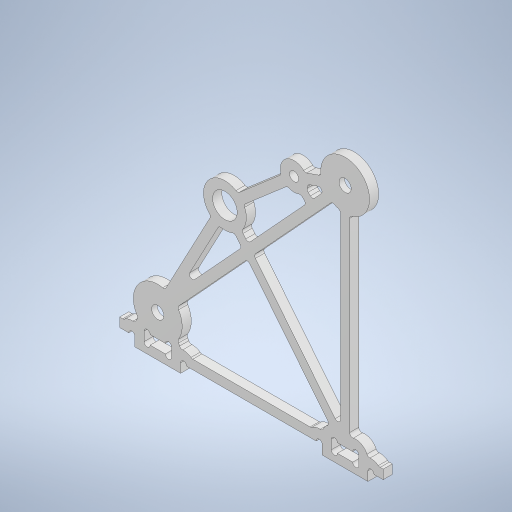
# Autodesk Inventor part: アーム 左フレーム
Saved by Autodesk Inventor 2023 (Build 270158000, 158)
## iProperties
Created: 2020-05-03
Part Number: アーム 左フレーム
Material: アルミニウム 2014-T6
Document SubType Name: Modeling
Designer: mozar
Density: 2.78927 g/cm^3
Appearance: サテン
Mass: 13.4791 g
Surface Area: 59.0115 cm^2
Volume: 4.83249 cm^3
Author: mozar
Autodesk Inventor part; units mm, degrees
(part 1 of 2)
ref_plane "YZ Plane" through (0, 0, 0) normal (1, 0, 0) x (0, 1, 0)
ref_plane "XZ Plane" through (0, 0, 0) normal (0, 1, 0) x (-1, 0, 0)
ref_plane "XY Plane" through (0, 0, 0) normal (0, 0, 1) x (1, 0, 0)
sketch "スケッチ1" plane through (0, 0, 0) normal (0, 0, 1) x (1, 0, 0)
  arc A0 (39.9627, 86.1428) -> (39.4448, 84.9887) centre (40.4104, 85.2486) ccw
  arc A1 (39.7226, 83.6386) -> (39.4448, 84.9887) centre (28.3399, 82) ccw
  arc A2 (39.7226, 83.6386) -> (40.6541, 82.7828) centre (40.7124, 83.7811) ccw
  line L0 (40.6541, 82.7828) -> (57.3541, 81.8067)
  arc A3 (57.3541, 81.8067) -> (58.3494, 82.4556) centre (57.4124, 82.805) ccw
  arc A4 (59.9805, 85.044) -> (58.3494, 82.4556) centre (65.3767, 79.8352) ccw
  arc A5 (59.9805, 85.044) -> (60.1364, 86.2219) centre (59.261, 85.7385) ccw
  line L1 (60.1364, 86.2219) -> (56.2648, 93.2331)
  arc A6 (56.2648, 93.2331) -> (54.9416, 93.6438) centre (55.3894, 92.7497) ccw
  line L2 (54.9416, 93.6438) -> (39.9627, 86.1428)
  arc A7 (62.7626, 87.6721) -> (63.8426, 87.1766) centre (63.638, 88.1555) ccw
  arc A8 (65.8023, 87.3231) -> (63.8426, 87.1766) centre (65.3767, 79.8352) ccw
  arc A9 (65.8023, 87.3231) -> (66.7965, 87.9737) centre (65.859, 88.3215) ccw
  line L3 (66.7965, 87.9737) -> (71.2039, 99.8518)
  arc A10 (71.2039, 99.8518) -> (69.8186, 101.0938) centre (70.2663, 100.1996) ccw
  line L4 (69.8186, 101.0938) -> (59.416, 95.8845)
  arc A11 (59.416, 95.8845) -> (58.9884, 94.5069) centre (59.8638, 94.9903) ccw
  line L5 (58.9884, 94.5069) -> (62.7626, 87.6721)
  arc A12 (68.6447, 103.8611) -> (68.5001, 105.7082) centre (68.197, 104.7553) ccw
  line L6 (68.5001, 105.7082) -> (51.8505, 111.0032)
  arc A13 (51.8505, 111.0032) -> (50.6721, 109.5669) centre (51.5475, 110.0503) ccw
  line L7 (50.6721, 109.5669) -> (56.5694, 98.8874)
  arc A14 (56.5694, 98.8874) -> (57.8925, 98.4767) centre (57.4448, 99.3708) ccw
  line L8 (57.8925, 98.4767) -> (68.6447, 103.8611)
  arc A15 (53.4182, 96.236) -> (53.8458, 97.6136) centre (52.9704, 97.1302) ccw
  line L9 (53.8458, 97.6136) -> (47.1934, 109.6604)
  arc A16 (47.1934, 109.6604) -> (45.4441, 109.6631) centre (46.318, 109.177) ccw
  line L10 (45.4441, 109.6631) -> (35.6044, 91.9739)
  arc A17 (35.6044, 91.9739) -> (35.8272, 90.7287) centre (36.4783, 91.4878) ccw
  arc A18 (37.3851, 89.1018) -> (35.8272, 90.7287) centre (28.3399, 82) ccw
  arc A19 (37.3851, 89.1018) -> (38.6194, 88.8252) centre (38.1716, 89.7194) ccw
  line L11 (38.6194, 88.8252) -> (53.4182, 96.236)
  circle A20 centre (28.3399, 82) radius 7.5
  circle A21 centre (74.8156, 105.2737) radius 1.5
  arc A22 (-14.025, 48) -> (-12.025, 48) centre (-13.025, 48) ccw
  line L12 (-12.025, 48) -> (-12.025, 51)
  arc A23 (-12.025, 51) -> (-14.025, 51) centre (-13.025, 51) ccw
  line L13 (-14.025, 51) -> (-19.025, 51)
  arc A24 (-19.025, 51) -> (-21.025, 51) centre (-20.025, 51) ccw
  line L14 (-21.025, 51) -> (-21.025, 48)
  arc A25 (-21.025, 48) -> (-19.025, 48) centre (-20.025, 48) ccw
  line L15 (-19.025, 48) -> (-14.025, 48)
  arc A26 (60.3767, 48) -> (62.3767, 48) centre (61.3767, 48) ccw
  line L16 (62.3767, 48) -> (62.3767, 51)
  arc A27 (62.3767, 51) -> (60.3767, 51) centre (61.3767, 51) ccw
  line L17 (60.3767, 51) -> (55.3767, 51)
  arc A28 (55.3767, 51) -> (53.3767, 51) centre (54.3767, 51) ccw
  line L18 (53.3767, 51) -> (53.3767, 48)
  arc A29 (53.3767, 48) -> (55.3767, 48) centre (54.3767, 48) ccw
  line L19 (55.3767, 48) -> (60.3767, 48)
  arc A30 (43.4972, 112.3347) -> (43.549, 113.1991) centre (42.6234, 112.8208) ccw
  arc A31 (43.3678, 113.8351) -> (43.549, 113.1991) centre (46.326, 114.3342) ccw
  arc A32 (43.3678, 113.8351) -> (42.8681, 114.5425) centre (42.3817, 113.6687) ccw
  line L20 (42.8681, 114.5425) -> (33.2246, 119.9111)
  arc A33 (33.2246, 119.9111) -> (32.0339, 119.7474) centre (32.7382, 119.0374) ccw
  arc A34 (28.9631, 117.8488) -> (32.0339, 119.7474) centre (26.4001, 125.4272) ccw
  arc A35 (28.9631, 117.8488) -> (28.2844, 116.8569) centre (29.2834, 116.9015) ccw
  line L21 (28.2844, 116.8569) -> (29.2919, 94.3022)
  arc A36 (29.2919, 94.3022) -> (30.1348, 93.3591) centre (30.2909, 94.3468) ccw
  arc A37 (31.8073, 92.9648) -> (30.1348, 93.3591) centre (28.3399, 82) ccw
  arc A38 (31.8073, 92.9648) -> (32.9827, 93.4322) centre (32.1088, 93.9183) ccw
  line L22 (32.9827, 93.4322) -> (43.4972, 112.3347)
  arc A39 (69.6092, 86.93) -> (69.9385, 85.7884) centre (70.5467, 86.5822) ccw
  arc A40 (72.822, 80.7396) -> (69.9385, 85.7884) centre (65.3767, 79.8352) ccw
  arc A41 (72.822, 80.7396) -> (73.638, 79.876) centre (73.8147, 80.8602) ccw
  line L23 (73.638, 79.876) -> (87.0818, 77.4622)
  arc A42 (87.0818, 77.4622) -> (88.1269, 78.9424) centre (87.2585, 78.4465) ccw
  line L24 (88.1269, 78.9424) -> (76.1666, 99.8838)
  arc A43 (76.1666, 99.8838) -> (74.3607, 99.7357) centre (75.2982, 99.3878) ccw
  line L25 (74.3607, 99.7357) -> (69.6092, 86.93)
  arc A44 (73.1078, 76.9232) -> (72.0424, 76.3973) centre (72.9311, 75.9389) ccw
  arc A45 (67.5826, 72.667) -> (72.0424, 76.3973) centre (65.3767, 79.8352) ccw
  arc A46 (67.5826, 72.667) -> (66.8767, 71.7112) centre (67.8767, 71.7112) ccw
  line L26 (66.8767, 71.7112) -> (66.8767, 58.0524)
  arc A47 (66.8767, 58.0524) -> (68.5183, 57.2854) centre (67.8767, 58.0524) ccw
  line L27 (68.5183, 57.2854) -> (87.0165, 72.7581)
  arc A48 (87.0165, 72.7581) -> (86.5516, 74.5094) centre (86.3749, 73.5252) ccw
  line L28 (86.5516, 74.5094) -> (73.1078, 76.9232)
  arc A49 (-29.708, 65.4922) -> (-29.5215, 64.3049) centre (-28.8251, 65.0226) ccw
  arc A50 (-28.6541, 63.3116) -> (-29.5215, 64.3049) centre (-35.0928, 58.5637) ccw
  arc A51 (-28.6541, 63.3116) -> (-27.5026, 62.9671) centre (-27.8492, 63.9051) ccw
  line L29 (-27.5026, 62.9671) -> (-4.985, 71.2866)
  arc A52 (-4.985, 71.2866) -> (-4.395, 72.5749) centre (-5.3316, 72.2246) ccw
  line L30 (-4.395, 72.5749) -> (-11.0543, 90.3814)
  arc A53 (-11.0543, 90.3814) -> (-12.0966, 91.0255) centre (-11.9909, 90.0311) ccw
  arc A54 (-15.1677, 91.227) -> (-12.0966, 91.0255) centre (-13.05, 100) ccw
  arc A55 (-15.1677, 91.227) -> (-16.2852, 90.7245) centre (-15.4023, 90.2549) ccw
  line L31 (-16.2852, 90.7245) -> (-29.708, 65.4922)
  arc A56 (-4.1377, 98.5784) -> (-3.549, 97.5038) centre (-3.1501, 98.4209) ccw
  line L32 (-3.549, 97.5038) -> (17.7068, 88.2599)
  arc A57 (17.7068, 88.2599) -> (18.9244, 88.6028) centre (18.1056, 89.177) ccw
  arc A58 (21.267, 91.0677) -> (18.9244, 88.6028) centre (28.3399, 82) ccw
  arc A59 (21.267, 91.0677) -> (21.5476, 92.3011) centre (20.652, 91.8562) ccw
  line L33 (21.5476, 92.3011) -> (10.495, 114.5492)
  arc A60 (10.495, 114.5492) -> (9.6102, 115.1042) centre (9.5994, 114.1043) ccw
  arc A61 (7.9613, 115.4364) -> (9.6102, 115.1042) centre (9.6587, 119.604) ccw
  arc A62 (7.9613, 115.4364) -> (6.9306, 115.2672) centre (7.5841, 114.5103) ccw
  line L34 (6.9306, 115.2672) -> (-4.721, 105.2086)
  arc A63 (-4.721, 105.2086) -> (-4.9636, 104.0076) centre (-4.0676, 104.4516) ccw
  arc A64 (-4.1377, 98.5784) -> (-4.9636, 104.0076) centre (-13.05, 100) ccw
  circle A65 centre (65.3767, 52.702) radius 1.5
  arc A66 (-24.6969, 51.9865) -> (-27.425, 51.2) centre (-25.025, 48) ccw
  arc A67 (-24.6969, 51.9865) -> (-23.6969, 52.5865) centre (-24.6149, 52.9832) ccw
  arc A68 (-22.7265, 53.9499) -> (-23.6969, 52.5865) centre (-20.025, 51) ccw
  arc A69 (-22.7265, 53.9499) -> (-23.2864, 55.6807) centre (-23.4019, 54.6874) ccw
  line L35 (-23.2864, 55.6807) -> (-26.6781, 56.0751)
  arc A70 (-26.6781, 56.0751) -> (-27.7157, 55.4687) centre (-26.7936, 55.0818) ccw
  arc A71 (-29.6192, 52.7293) -> (-27.7157, 55.4687) centre (-35.0928, 58.5637) ccw
  arc A72 (-29.6192, 52.7293) -> (-28.935, 51) centre (-28.935, 52) ccw
  line L36 (-28.935, 51) -> (-28.025, 51)
  arc A73 (-28.025, 51) -> (-27.425, 51.2) centre (-28.025, 52) ccw
  circle A74 centre (4.1532, 54) radius 1.5
  circle A75 centre (-35.0928, 58.5637) radius 4
  arc A76 (-6.2073, 53.6947) -> (-6.6633, 51.7611) centre (-6.3229, 52.7014) ccw
  arc A77 (-5.625, 51.2) -> (-6.6633, 51.7611) centre (-8.025, 48) ccw
  arc A78 (-5.625, 51.2) -> (-5.025, 51) centre (-5.025, 52) ccw
  line L37 (-5.025, 51) -> (-0.2915, 51)
  arc A79 (-0.2915, 51) -> (-0.176, 52.9933) centre (-0.2915, 52) ccw
  line L38 (-0.176, 52.9933) -> (-6.2073, 53.6947)
  circle A80 centre (-42.5549, 50.4818) radius 1.5
  circle A81 centre (92.0829, 75.0403) radius 1.5
  circle A82 centre (34.927, 132.3764) radius 1.5
  circle A83 centre (26.4001, 125.4272) radius 4
  arc A84 (38.4894, 120.4137) -> (39.8212, 121.8216) centre (38.9758, 121.2874) ccw
  line L39 (39.8212, 121.8216) -> (36.0614, 127.7726)
  arc A85 (36.0614, 127.7726) -> (34.2364, 127.0372) centre (35.216, 127.2385) ccw
  arc A86 (34.1958, 123.6306) -> (34.2364, 127.0372) centre (26.4001, 125.4272) ccw
  arc A87 (34.1958, 123.6306) -> (34.6838, 122.5323) centre (35.1702, 123.406) ccw
  line L40 (34.6838, 122.5323) -> (38.4894, 120.4137)
  circle A88 centre (46.326, 114.3342) radius 1.5
  arc A89 (68.7767, 51.2) -> (68.7327, 51.2326) centre (66.3767, 48) ccw
  arc A90 (68.7767, 51.2) -> (69.3767, 51) centre (69.3767, 52) ccw
  line L41 (69.3767, 51) -> (77.3767, 51)
  arc A91 (77.3767, 51) -> (78.3767, 52) centre (77.3767, 52) ccw
  line L42 (78.3767, 52) -> (78.3767, 59.4801)
  arc A92 (78.3767, 59.4801) -> (76.7351, 60.2472) centre (77.3767, 59.4801) ccw
  line L43 (76.7351, 60.2472) -> (68.7342, 53.5548)
  arc A93 (68.7342, 53.5548) -> (68.376, 52.7664) centre (69.3758, 52.7878) ccw
  arc A94 (68.3354, 52.206) -> (68.376, 52.7664) centre (65.3767, 52.702) ccw
  arc A95 (68.3354, 52.206) -> (68.7327, 51.2326) centre (69.3217, 52.0407) ccw
  arc A96 (-24.7713, 60.778) -> (-24.5402, 58.8467) centre (-24.4247, 59.84) ccw
  line L44 (-24.5402, 58.8467) -> (0.2632, 55.9625)
  arc A97 (0.2632, 55.9625) -> (1.3153, 57.3061) centre (0.3787, 56.9558) ccw
  line L45 (1.3153, 57.3061) -> (-2.6435, 67.8917)
  arc A98 (-2.6435, 67.8917) -> (-3.9267, 68.4794) centre (-3.5802, 67.5414) ccw
  line L46 (-3.9267, 68.4794) -> (-24.7713, 60.778)
  arc A99 (-7.8805, 92.6022) -> (-8.2443, 91.4322) centre (-7.3077, 91.7825) ccw
  line L47 (-8.2443, 91.4322) -> (-1.5781, 73.6072)
  arc A100 (-1.5781, 73.6072) -> (-0.2949, 73.0195) centre (-0.6415, 73.9575) ccw
  line L48 (-0.2949, 73.0195) -> (16.3317, 79.1624)
  arc A101 (16.3317, 79.1624) -> (16.9735, 80.2524) centre (15.9851, 80.1005) ccw
  arc A102 (17.0899, 84.3844) -> (16.9735, 80.2524) centre (28.3399, 82) ccw
  arc A103 (17.0899, 84.3844) -> (16.5104, 85.5088) centre (16.1116, 84.5918) ccw
  line L49 (16.5104, 85.5088) -> (-4.7454, 94.7527)
  arc A104 (-4.7454, 94.7527) -> (-5.9328, 94.4506) centre (-5.1442, 93.8357) ccw
  arc A105 (-7.8805, 92.6022) -> (-5.9328, 94.4506) centre (-13.05, 100) ccw
  arc A106 (18.5677, 75.9375) -> (17.3714, 76.3484) centre (17.718, 75.4104) ccw
  line L50 (17.3714, 76.3484) -> (0.7634, 70.2123)
  arc A107 (0.7634, 70.2123) -> (0.1733, 68.924) centre (1.11, 69.2743) ccw
  line L51 (0.1733, 68.924) -> (4.0811, 58.475)
  arc A108 (4.0811, 58.475) -> (5.7745, 58.1716) centre (5.0177, 58.8253) ccw
  line L52 (5.7745, 58.1716) -> (19.1987, 73.7122)
  arc A109 (19.1987, 73.7122) -> (19.2338, 74.9766) centre (18.4419, 74.3659) ccw
  arc A110 (18.5677, 75.9375) -> (19.2338, 74.9766) centre (28.3399, 82) ccw
  arc A111 (22.7149, 71.9696) -> (21.469, 71.7511) centre (22.2257, 71.0974) ccw
  line L53 (21.469, 71.7511) -> (7.3295, 55.3824)
  arc A112 (7.3295, 55.3824) -> (7.103, 54.5465) centre (8.0862, 54.7287) ccw
  arc A113 (6.7512, 52.5) -> (7.103, 54.5465) centre (4.1532, 54) ccw
  arc A114 (6.7512, 52.5) -> (7.6173, 51) centre (7.6173, 52) ccw
  line L54 (7.6173, 51) -> (25.8399, 51)
  arc A115 (25.8399, 51) -> (26.8399, 52) centre (25.8399, 52) ccw
  line L55 (26.8399, 52) -> (26.8399, 69.7526)
  arc A116 (26.8399, 69.7526) -> (26.0399, 70.7323) centre (25.8399, 69.7526) ccw
  arc A117 (22.7149, 71.9696) -> (26.0399, 70.7323) centre (28.3399, 82) ccw
  arc A118 (30.6399, 70.7323) -> (29.8399, 69.7526) centre (30.8399, 69.7526) ccw
  line L56 (29.8399, 69.7526) -> (29.8399, 52)
  arc A119 (29.8399, 52) -> (30.8399, 51) centre (30.8399, 52) ccw
  line L57 (30.8399, 51) -> (46.3767, 51)
  arc A120 (46.3767, 51) -> (46.9767, 51.2) centre (46.3767, 52) ccw
  arc A121 (49.7048, 51.9865) -> (46.9767, 51.2) centre (49.3767, 48) ccw
  arc A122 (49.7048, 51.9865) -> (50.7048, 52.5865) centre (49.7868, 52.9832) ccw
  arc A123 (56.7767, 54.2) -> (50.7048, 52.5865) centre (54.3767, 51) ccw
  arc A124 (56.7767, 54.2) -> (57.3767, 54) centre (57.3767, 55) ccw
  line L58 (57.3767, 54) -> (58.3767, 54)
  arc A125 (58.3767, 54) -> (58.9767, 54.2) centre (58.3767, 55) ccw
  arc A126 (59.0037, 54.2201) -> (58.9767, 54.2) centre (61.3767, 51) ccw
  arc A127 (59.0037, 54.2201) -> (59.0309, 55.8094) centre (58.4105, 55.0251) ccw
  line L59 (59.0309, 55.8094) -> (37.0148, 73.2252)
  arc A128 (37.0148, 73.2252) -> (35.75, 73.2056) centre (36.3944, 72.4409) ccw
  arc A129 (30.6399, 70.7323) -> (35.75, 73.2056) centre (28.3399, 82) ccw
  arc A130 (25.5394, 93.1538) -> (26.2949, 94.1683) centre (25.2959, 94.1237) ccw
  line L60 (26.2949, 94.1683) -> (25.2874, 116.723)
  arc A131 (25.2874, 116.723) -> (24.5231, 117.6505) centre (24.2884, 116.6784) ccw
  arc A132 (19.8716, 120.8035) -> (24.5231, 117.6505) centre (26.4001, 125.4272) ccw
  arc A133 (19.8716, 120.8035) -> (18.727, 121.17) centre (19.0555, 120.2256) ccw
  line L61 (18.727, 121.17) -> (14.7786, 119.7967)
  arc A134 (14.7786, 119.7967) -> (14.1165, 118.9889) centre (15.1071, 118.8522) ccw
  arc A135 (13.2739, 116.9243) -> (14.1165, 118.9889) centre (9.6587, 119.604) ccw
  arc A136 (13.2739, 116.9243) -> (13.1817, 115.8839) centre (14.0773, 116.3288) ccw
  line L62 (13.1817, 115.8839) -> (24.2343, 93.6359)
  arc A137 (24.2343, 93.6359) -> (25.3867, 93.1143) centre (25.1298, 94.0808) ccw
  arc A138 (25.5394, 93.1538) -> (25.3867, 93.1143) centre (28.3399, 82) ccw
  arc A139 (16.6463, 125.18) -> (18.408, 125.7823) centre (17.409, 125.8267) ccw
  arc A140 (30.493, 132.3009) -> (18.408, 125.7823) centre (26.4001, 125.4272) ccw
  arc A141 (30.493, 132.3009) -> (31.9852, 132.9642) centre (31.0046, 133.1602) ccw
  arc A142 (37.763, 131.3981) -> (31.9852, 132.9642) centre (34.927, 132.3764) ccw
  arc A143 (37.763, 131.3981) -> (37.8629, 130.5378) centre (38.7083, 131.0719) ccw
  line L63 (37.8629, 130.5378) -> (45.9263, 117.7752)
  arc A144 (45.9263, 117.7752) -> (46.6603, 117.3156) centre (46.7717, 118.3093) ccw
  arc A145 (49.126, 115.4113) -> (46.6603, 117.3156) centre (46.326, 114.3342) ccw
  arc A146 (49.126, 115.4113) -> (49.7562, 114.8174) centre (50.0593, 115.7703) ccw
  line L64 (49.7562, 114.8174) -> (72.2946, 107.6495)
  arc A147 (72.2946, 107.6495) -> (73.1521, 107.7703) centre (72.5976, 108.6025) ccw
  arc A148 (77.6052, 104.17) -> (73.1521, 107.7703) centre (74.8156, 105.2737) ccw
  arc A149 (77.6052, 104.17) -> (77.6667, 103.3062) centre (78.5351, 103.8022) ccw
  line L65 (77.6667, 103.3062) -> (91.8368, 78.4957)
  arc A150 (91.8368, 78.4957) -> (92.5496, 78.0038) centre (92.7052, 78.9916) ccw
  arc A151 (91.4896, 72.0996) -> (92.5496, 78.0038) centre (92.0829, 75.0403) ccw
  arc A152 (91.4896, 72.0996) -> (90.6502, 71.8864) centre (91.2918, 71.1193) ccw
  line L66 (90.6502, 71.8864) -> (81.7351, 64.4294)
  arc A153 (81.7351, 64.4294) -> (81.3767, 63.6624) centre (82.3767, 63.6624) ccw
  line L67 (81.3767, 63.6624) -> (81.3767, 48)
  line L68 (81.3767, 48) -> (67.3767, 48)
  arc A154 (67.3767, 48) -> (65.3767, 48) centre (66.3767, 48) ccw
  line L69 (65.3767, 48) -> (65.3767, 45)
  line L70 (65.3767, 45) -> (50.3767, 45)
  line L71 (50.3767, 45) -> (50.3767, 48)
  arc A155 (50.3767, 48) -> (48.3767, 48) centre (49.3767, 48) ccw
  line L72 (48.3767, 48) -> (-7.025, 48)
  arc A156 (-7.025, 48) -> (-9.025, 48) centre (-8.025, 48) ccw
  line L73 (-9.025, 48) -> (-9.025, 45)
  line L74 (-9.025, 45) -> (-24.025, 45)
  line L75 (-24.025, 45) -> (-24.025, 48)
  arc A157 (-24.025, 48) -> (-26.025, 48) centre (-25.025, 48) ccw
  line L76 (-26.025, 48) -> (-40.586, 48)
  arc A158 (-40.586, 48) -> (-41.0782, 47.8705) centre (-40.586, 47) ccw
  arc A159 (-42.9601, 53.4544) -> (-41.0782, 47.8705) centre (-42.5549, 50.4818) ccw
  arc A160 (-42.9601, 53.4544) -> (-42.206, 54.9028) centre (-43.0951, 54.4452) ccw
  arc A161 (-36.1143, 66.4982) -> (-42.206, 54.9028) centre (-35.0928, 58.5637) ccw
  arc A162 (-36.1143, 66.4982) -> (-35.6612, 68.3041) centre (-36.242, 67.49) ccw
  arc A163 (16.6463, 125.18) -> (-35.6612, 68.3041) centre (-13.05, 100) ccw
  arc A164 (58.092, 78.0514) -> (57.179, 78.8118) centre (57.1207, 77.8135) ccw
  line L77 (57.179, 78.8118) -> (40.479, 79.7879)
  arc A165 (40.479, 79.7879) -> (39.4542, 79.0465) centre (40.4207, 78.7896) ccw
  arc A166 (38.6039, 76.8133) -> (39.4542, 79.0465) centre (28.3399, 82) ccw
  arc A167 (38.6039, 76.8133) -> (38.876, 75.578) centre (39.4964, 76.3623) ccw
  line L78 (38.876, 75.578) -> (62.2563, 57.083)
  arc A168 (62.2563, 57.083) -> (63.8767, 57.8673) centre (62.8767, 57.8673) ccw
  line L79 (63.8767, 57.8673) -> (63.8767, 71.7112)
  arc A169 (63.8767, 71.7112) -> (63.1709, 72.667) centre (62.8767, 71.7112) ccw
  arc A170 (58.092, 78.0514) -> (63.1709, 72.667) centre (65.3767, 79.8352) ccw
  circle A171 centre (65.3767, 79.8352) radius 4.5
  arc A172 (-21.9546, 98.5311) -> (-22.8529, 99.3644) centre (-22.9413, 98.3683) ccw
  line L80 (-22.8529, 99.3644) -> (-47.8911, 101.5872)
  arc A173 (-47.8911, 101.5872) -> (-48.9794, 100.608) centre (-47.9795, 100.5911) ccw
  arc A174 (-48.9794, 100.608) -> (-32.1537, 69.5642) centre (-13.05, 100) ccw
  arc A175 (-32.1537, 69.5642) -> (-30.7392, 69.9415) centre (-31.622, 70.4111) ccw
  line L81 (-30.7392, 69.9415) -> (-18.9338, 92.1335)
  arc A176 (-18.9338, 92.1335) -> (-19.1416, 93.341) centre (-19.8166, 92.6031) ccw
  arc A177 (-21.9546, 98.5311) -> (-19.1416, 93.341) centre (-13.05, 100) ccw
  arc A178 (-17.8733, 107.628) -> (-17.4559, 108.78) centre (-18.4077, 108.4732) ccw
  line L82 (-17.4559, 108.78) -> (-25.1673, 132.7046)
  arc A179 (-25.1673, 132.7046) -> (-26.4932, 133.3253) centre (-26.1191, 132.3979) ccw
  arc A180 (-26.4932, 133.3253) -> (-48.5246, 105.731) centre (-13.05, 100) ccw
  arc A181 (-48.5246, 105.731) -> (-47.6258, 104.5754) centre (-47.5374, 105.5715) ccw
  line L83 (-47.6258, 104.5754) -> (-22.5876, 102.3526)
  arc A182 (-22.5876, 102.3526) -> (-21.5566, 103.0147) centre (-22.4992, 103.3487) ccw
  arc A183 (-17.8733, 107.628) -> (-21.5566, 103.0147) centre (-13.05, 100) ccw
  arc A184 (11.2534, 123.8119) -> (12.3137, 125.4554) centre (11.6078, 124.747) ccw
  arc A185 (12.3137, 125.4554) -> (-21.598, 134.903) centre (-13.05, 100) ccw
  arc A186 (-21.598, 134.903) -> (-22.3119, 133.625) centre (-21.3602, 133.9317) ccw
  line L84 (-22.3119, 133.625) -> (-14.6006, 109.7003)
  arc A187 (-14.6006, 109.7003) -> (-13.5891, 109.0089) centre (-13.6488, 110.0071) ccw
  arc A188 (-7.905, 107.4148) -> (-13.5891, 109.0089) centre (-13.05, 100) ccw
  arc A189 (-7.905, 107.4148) -> (-6.6814, 107.4795) centre (-7.3349, 108.2364) ccw
  line L85 (-6.6814, 107.4795) -> (4.9702, 117.5381)
  arc A190 (4.9702, 117.5381) -> (5.288, 118.533) centre (4.3167, 118.295) ccw
  arc A191 (11.2534, 123.8119) -> (5.288, 118.533) centre (9.6587, 119.604) ccw
  circle A192 centre (9.6587, 119.604) radius 1.5
  circle A193 centre (-13.05, 100) radius 4.025
  circle A194 centre (-13.05, 100) radius 7.025
  circle A195 centre (-35.0928, 58.5637) radius 8
  circle A196 centre (26.4001, 125.4272) radius 8
  circle A197 centre (9.6587, 119.604) radius 4.5
  line L86 (-35.0928, 58.5637) -> (-13.05, 100) construction
  line L87 (-33.7685, 57.8592) -> (-11.7257, 99.2955)
  line L88 (-14.3743, 100.7045) -> (-36.4171, 59.2682)
  arc A198 (-36.4171, 59.2682) -> (-33.7685, 57.8592) centre (-35.0928, 58.5637) ccw
  arc A199 (-11.7257, 99.2955) -> (-14.3743, 100.7045) centre (-13.05, 100) ccw
  line L89 (-13.05, 100) -> (9.6587, 119.604) construction
  line L90 (-12.0698, 98.8646) -> (10.6389, 118.4685)
  line L91 (8.6785, 120.7394) -> (-14.0302, 101.1354)
  arc A200 (-14.0302, 101.1354) -> (-12.0698, 98.8646) centre (-13.05, 100) ccw
  arc A201 (10.6389, 118.4685) -> (8.6785, 120.7394) centre (9.6587, 119.604) ccw
  line L92 (9.6587, 119.604) -> (26.4001, 125.4272) construction
  line L93 (10.1515, 118.1872) -> (26.8929, 124.0104)
  line L94 (25.9073, 126.8439) -> (9.1659, 121.0207)
  arc A202 (9.1659, 121.0207) -> (10.1515, 118.1872) centre (9.6587, 119.604) ccw
  arc A203 (26.8929, 124.0104) -> (25.9073, 126.8439) centre (26.4001, 125.4272) ccw
  line L95 (26.4001, 125.4272) -> (-35.0928, 58.5637) construction
  line L96 (25.296, 126.4426) -> (-36.1968, 59.5791)
  line L97 (-33.9887, 57.5483) -> (27.5042, 124.4118)
  arc A204 (27.5042, 124.4118) -> (25.296, 126.4426) centre (26.4001, 125.4272) ccw
  arc A205 (-36.1968, 59.5791) -> (-33.9887, 57.5483) centre (-35.0928, 58.5637) ccw
  point P0 (0, 0)
  point P1 (0, 0)
  point P2 (-24.0714, 79.2818)
  point P3 (-1.6956, 109.802)
  point P4 (18.0294, 122.5156)
  point P5 (-4.3463, 91.9954)
  point P6 (-14.9489, 93.2365)
  point P7 (-6.8748, 103.3493)
  point P8 (6.9306, 115.2672)
  point P9 (7.4274, 115.6961)
  point P10 (7.9613, 115.4364)
  point P11 (13.2739, 116.9243)
  point P12 (14.1586, 119.581)
  point P13 (18.727, 121.17)
  point P14 (19.471, 121.4288)
  point P15 (19.9767, 120.6586)
  point P16 (-28.2664, 68.2022)
  point P17 (5.467, 117.967)
  point P18 (-6.6814, 107.4795)
  point P19 (-8.8352, 105.6202)
  point P20 (-17.5975, 94.6455)
  point P21 (-30.7392, 69.9415)
  point P22 (-32.7265, 66.2057)
  point P23 (-28.6541, 63.3116)
  point P24 (-28.6693, 63.3323)
  point P25 (22.1848, 118.6278)
  point P26 (24.5231, 117.6505)
  point P27 (34.1958, 123.6306)
  point P28 (34.2364, 127.0372)
  point P29 (18.4854, 124.2623)
  point P30 (13.1731, 122.4145)
  dimension "d0" = 3
  dimension "d1" = 3
  dimension "d2" = 3
  dimension "d3" = 3
  dimension "d4" = 3
  constraints: 378 point on circle, 204 end point, 203 centre point, 16 tangent, 15 horizontal, 14 vertical, 4 midpoint, 4 parallel, 3 coincident, 1 concentric, 723 other
  measures "d0" radial gap between concentric circles of A193 A194
  measures "d1" diameter of A199
  measures "d2" diameter of A201
  measures "d3" diameter of A203
  measures "d4" diameter of A205
extrude "押し出し1" add sketch "スケッチ1" against normal blind 3 contours A34 A196 A132 L97 A83 L94 A140 A86 | L97 L62 L96 A132 | A132 L96 L93 A83 L97 | A132 A196 L93 L96 | L97 L33 L96 L62 | L97 A203 L94 A83 | A83 L93 A203 L97 | L96 A83 L93 | L93 A196 L94 A83 L96 | L97 L32 L96 L33 | A83 L96 A204 A203 L93 | L61 L93 A197 L94 A196 | A83 L94 A204 L96 | L97 L49 L96 L32 | A197 A61 L90 L93 A135 | L97 L47 L96 L49 | L94 A192 L91 A197 A191 | A197 L93 L90 A192 L94 | L97 L30 L96 L47 | A195 L88 A75 L97 A50 A71 A161 | A192 | L93 A192 L90 | L90 A197 L91 A192 L93 | L97 A50 A49 L31 L96 L30 | L88 L81 A194 L87 L31 L96 A195 | A195 L96 A75 L88 | L90 L34 A194 L91 L85 A197 | L97 A75 L87 A195 A50 | L96 L31 L87 A195 | A195 L87 A75 L96 | L88 A198 L97 A75 | A75 L96 A205 L88 | A195 L87 A49 | L97 A198 L87 A75 | A75 L87 A198 A205 L96 | L90 A193 L91 A194 | A194 L87 A193 L90 | L88 A193 L87 A194 | A194 L91 A193 L88 | L90 L87 A199 L91 A193 | A193 L87 L90 | L88 A200 L90 L87 A193 | A193 L91 A199 L88 | L90 A200 A199 L87
hole "穴1" at (9.6587, 119.604, 0) direction (0, 0, -1) diameter 3 depth 12 tip angle 118
hole "穴2" at (-13.05, 100, 0) direction (0, 0, -1) diameter 8.05 depth 12 tip angle 118
hole "穴3" at (26.4001, 125.4272, 0) at (-35.0928, 58.5637, 0) direction (0, 0, -1) diameter 4 depth 12 tip angle 118
sketch "スケッチ2" plane through (0, 0, -3) normal (0, 0, -1) x (-1, 0, 0)
  circle A0 centre (-26.4001, 125.4272) radius 2 projected
  circle A1 centre (35.0928, 58.5637) radius 2 projected
  circle A2 centre (13.05, 100) radius 4.025 projected
  circle A3 centre (-9.6587, 119.604) radius 1.5 projected
  arc A4 (6.8748, 103.3493) -> (14.9489, 93.2365) centre (13.05, 100) ccw projected
  line L0 (6.8748, 103.3493) -> (-7.4274, 115.6961) projected
  arc A5 (-14.1586, 119.581) -> (-7.4274, 115.6961) centre (-9.6587, 119.604) ccw projected
  line L1 (-14.1586, 119.581) -> (-19.471, 121.4288) projected
  arc A6 (-19.9767, 120.6586) -> (-19.471, 121.4288) centre (-26.4001, 125.4272) ccw projected
  line L2 (-19.9767, 120.6586) -> (28.2664, 68.2022) projected
  line L3 (28.2664, 68.2022) -> (14.9489, 93.2365) projected
  line L4 (-5.467, 117.967) -> (8.8352, 105.6202) projected
  arc A7 (17.5975, 94.6455) -> (8.8352, 105.6202) centre (13.05, 100) ccw projected
  line L5 (17.5975, 94.6455) -> (32.7265, 66.2057) projected
  arc A8 (28.6693, 63.3323) -> (32.7265, 66.2057) centre (35.0928, 58.5637) ccw projected
  line L6 (28.6693, 63.3323) -> (-22.1848, 118.6278) projected
  arc A9 (-18.4854, 124.2623) -> (-22.1848, 118.6278) centre (-26.4001, 125.4272) ccw projected
  line L7 (-18.4854, 124.2623) -> (-13.1731, 122.4145) projected
  arc A10 (-5.467, 117.967) -> (-13.1731, 122.4145) centre (-9.6587, 119.604) ccw projected
  circle A11 centre (35.0928, 58.5637) radius 4
  circle A12 centre (-26.4001, 125.4272) radius 2 projected
  circle A13 centre (-26.4001, 125.4272) radius 4
  point P0 (0, 0)
  dimension "d28" = 8
  dimension "d29" = 8
  constraints: 2 centre point, 2 coincident
  measures "d28" diameter of A11
  measures "d29" diameter of A13
extrude "押し出し2" cut sketch "スケッチ2" against normal blind 0.7 contours A0 | A1 | A11 | A13
sketch "スケッチ3" plane through (0, 0, -3) normal (0, 0, -1) x (-1, 0, 0)
  circle A0 centre (35.0928, 58.5637) radius 4 projected
  circle A1 centre (-26.4001, 125.4272) radius 4 projected
  circle A2 centre (13.05, 100) radius 4.025 projected
  circle A3 centre (-9.6587, 119.604) radius 1.5 projected
  arc A4 (6.8748, 103.3493) -> (14.9489, 93.2365) centre (13.05, 100) ccw projected
  line L0 (6.8748, 103.3493) -> (-7.4274, 115.6961) projected
  arc A5 (-14.1586, 119.581) -> (-7.4274, 115.6961) centre (-9.6587, 119.604) ccw projected
  line L1 (-14.1586, 119.581) -> (-19.471, 121.4288) projected
  arc A6 (-19.9767, 120.6586) -> (-19.471, 121.4288) centre (-26.4001, 125.4272) ccw projected
  line L2 (-19.9767, 120.6586) -> (28.2664, 68.2022) projected
  line L3 (28.2664, 68.2022) -> (14.9489, 93.2365) projected
  line L4 (-5.467, 117.967) -> (8.8352, 105.6202) projected
  arc A7 (17.5975, 94.6455) -> (8.8352, 105.6202) centre (13.05, 100) ccw projected
  line L5 (17.5975, 94.6455) -> (32.7265, 66.2057) projected
  arc A8 (28.6693, 63.3323) -> (32.7265, 66.2057) centre (35.0928, 58.5637) ccw projected
  line L6 (28.6693, 63.3323) -> (-22.1848, 118.6278) projected
  arc A9 (-18.4854, 124.2623) -> (-22.1848, 118.6278) centre (-26.4001, 125.4272) ccw projected
  line L7 (-18.4854, 124.2623) -> (-13.1731, 122.4145) projected
  arc A10 (-5.467, 117.967) -> (-13.1731, 122.4145) centre (-9.6587, 119.604) ccw projected
  circle A11 centre (13.05, 100) radius 4.025 projected
  line L8 (13.05, 100) -> (5.4504, 93.0108) construction
  line L9 (28.2664, 68.2022) -> (-19.9767, 120.6586) projected
  line L10 (12.0346, 101.1041) -> (4.435, 94.1149)
  line L11 (6.4658, 91.9067) -> (14.0654, 98.8959)
  arc A12 (14.0654, 98.8959) -> (12.0346, 101.1041) centre (13.05, 100) ccw
  arc A13 (4.435, 94.1149) -> (6.4658, 91.9067) centre (5.4504, 93.0108) ccw
  line L12 (-9.6587, 119.604) -> (-14.7232, 114.9463) construction
  line L13 (-10.6741, 120.708) -> (-15.7386, 116.0504)
  line L14 (-13.7078, 113.8422) -> (-8.6433, 118.4999)
  arc A14 (-8.6433, 118.4999) -> (-10.6741, 120.708) centre (-9.6587, 119.604) ccw
  arc A15 (-15.7386, 116.0504) -> (-13.7078, 113.8422) centre (-14.7232, 114.9463) ccw
  point P0 (0, 0)
  point P1 (9.2502, 96.5054)
  point P2 (-12.1909, 117.2751)
  point P3 (9.0139, 94.2502)
  point P4 (6.9831, 96.4583)
  point P5 (-11.7661, 115.6279)
  point P6 (-13.7969, 117.8361)
  dimension "d33" = 3
  dimension "d34" = 3
  constraints: 16 end point, 8 point on circle, 8 tangent, 4 centre point, 2 midpoint, 2 parallel, 2 perpendicular, 2 point on line
  measures "d33" diameter of A13
  measures "d34" diameter of A15
extrude "押し出し3" add sketch "スケッチ3" against normal blind 3 contours L2 L13 A5 L14
fillet "フィレット1" radius 1 19 edges at (22.1848, 118.6278, -1.5) (19.9767, 120.6586, -1.5) (19.471, 121.4288, -1.5) (18.4854, 124.2623, -1.5) (13.1731, 122.4145, -1.5) (14.1586, 119.581, -1.5) (13.7969, 117.8361, -1.5) (15.7386, 116.0504, -1.5) (13.7078, 113.8422, -1.5) (11.7661, 115.6279, -1.5) (7.4274, 115.6961, -1.5) (5.467, 117.967, -1.5) (-6.8748, 103.3493, -1.5) (-8.8352, 105.6202, -1.5) (-14.9489, 93.2365, -1.5) (-17.5975, 94.6455, -1.5) (-28.2664, 68.2022, -1.5) (-32.7265, 66.2057, -1.5) (-28.6693, 63.3323, -1.5)
sketch "スケッチ4" plane through (0, 0, -3) normal (0, 0, -1) x (-1, 0, 0)
  line L0 (9.025, 45) -> (24.025, 45) projected
  line L1 (26.025, 48) -> (40.586, 48) projected
  arc A0 (28.2548, 62.7161) -> (28.1361, 63.912) centre (27.4001, 63.2351) ccw projected
  line L2 (28.1361, 63.912) -> (-21.6516, 118.048) projected
  arc A1 (-21.6516, 118.048) -> (-22.8335, 118.2662) centre (-22.3876, 117.3711) ccw projected
  arc A2 (-18.4115, 125.0013) -> (-22.8335, 118.2662) centre (-26.4001, 125.4272) ccw projected
  arc A3 (-18.4115, 125.0013) -> (-17.7414, 124.0035) centre (-17.4129, 124.948) ccw projected
  line L3 (-17.7414, 124.0035) -> (-13.793, 122.6301) projected
  arc A4 (-13.793, 122.6301) -> (-12.7725, 122.8527) centre (-13.4645, 123.5746) ccw projected
  arc A5 (-5.288, 118.533) -> (-12.7725, 122.8527) centre (-9.6587, 119.604) ccw projected
  arc A6 (-5.288, 118.533) -> (-4.9702, 117.5381) centre (-4.3167, 118.295) ccw projected
  line L4 (-4.9702, 117.5381) -> (8.2579, 106.1185) projected
  arc A7 (8.2579, 106.1185) -> (9.4271, 106.0187) centre (8.9114, 106.8755) ccw projected
  arc A8 (18.1172, 95.1344) -> (9.4271, 106.0187) centre (13.05, 100) ccw projected
  arc A9 (18.1172, 95.1344) -> (17.9557, 93.9721) centre (18.8385, 94.4418) ccw projected
  line L5 (17.9557, 93.9721) -> (32.3566, 66.9011) projected
  arc A10 (32.3566, 66.9011) -> (33.4453, 66.3922) centre (33.2394, 67.3708) ccw projected
  arc A11 (28.2548, 62.7161) -> (33.4453, 66.3922) centre (35.0928, 58.5637) ccw projected
  line L6 (-13.0309, 113.1062) -> (22.9794, 73.9509) projected
  arc A12 (22.9794, 73.9509) -> (24.5983, 75.0975) centre (23.7154, 74.6278) ccw projected
  line L7 (24.5983, 75.0975) -> (15.3071, 92.5632) projected
  arc A13 (15.3071, 92.5632) -> (14.253, 93.0788) centre (14.4242, 92.0935) ccw projected
  arc A14 (-11.2244, 115.3851) -> (-12.2492, 115.1836) centre (-11.5723, 114.4476) ccw projected
  line L8 (-12.2492, 115.1836) -> (-12.9717, 114.5191) projected
  arc A15 (-12.9717, 114.5191) -> (-13.0309, 113.1062) centre (-12.2948, 113.7831) ccw projected
  arc A16 (6.5669, 102.7056) -> (6.2975, 103.8477) centre (5.644, 103.0907) ccw projected
  line L9 (6.2975, 103.8477) -> (-6.9306, 115.2672) projected
  arc A17 (-6.9306, 115.2672) -> (-7.9613, 115.4364) centre (-7.5841, 114.5103) ccw projected
  arc A18 (-11.2244, 115.3851) -> (-7.9613, 115.4364) centre (-9.6587, 119.604) ccw projected
  arc A19 (-17.4982, 120.7426) -> (-18.5628, 119.1212) centre (-17.8267, 119.7981) ccw projected
  arc A20 (-16.4155, 116.7864) -> (-15.0025, 116.7273) centre (-15.6794, 117.4633) ccw projected
  line L10 (-15.0025, 116.7273) -> (-14.28, 117.3918) projected
  arc A21 (-14.28, 117.3918) -> (-13.9936, 118.3962) centre (-14.9569, 118.1278) ccw projected
  arc A22 (-14.1165, 118.9889) -> (-13.9936, 118.3962) centre (-9.6587, 119.604) ccw projected
  arc A23 (-14.1165, 118.9889) -> (-14.7786, 119.7967) centre (-15.1071, 118.8522) ccw projected
  line L11 (-14.7786, 119.7967) -> (-17.4982, 120.7426) projected
  circle A24 centre (35.0928, 58.5637) radius 4 projected
  circle A25 centre (-26.4001, 125.4272) radius 4 projected
  circle A26 centre (13.05, 100) radius 4.025 projected
  circle A27 centre (-9.6587, 119.604) radius 1.5 projected
  line L12 (12.025, 48) -> (12.025, 51) projected
  line L13 (21.025, 51) -> (21.025, 48) projected
  line L14 (24.025, 45) -> (24.025, 48) projected
  line L15 (9.025, 48) -> (9.025, 45) projected
  line L16 (27.5928, 48) -> (42.5928, 48)
  line L17 (42.5928, 48) -> (42.5928, 45)
  line L18 (42.5928, 45) -> (27.5928, 45)
  line L19 (27.5928, 45) -> (27.5928, 48)
  line L20 (32.5928, 48) -> (37.5928, 48)
  line L21 (39.5928, 48) -> (39.5928, 51)
  line L22 (37.5928, 51) -> (32.5928, 51)
  line L23 (30.5928, 51) -> (30.5928, 48)
  line L24 (35.0928, 51) -> (35.0928, 58.5637)
  arc A28 (32.5928, 51) -> (30.5928, 51) centre (31.5928, 51) ccw
  arc A29 (39.5928, 51) -> (37.5928, 51) centre (38.5928, 51) ccw
  arc A30 (30.5928, 48) -> (32.5928, 48) centre (31.5928, 48) ccw
  arc A31 (37.5928, 48) -> (39.5928, 48) centre (38.5928, 48) ccw
  line L25 (27.5928, 48) -> (27.5928, 51)
  arc A32 (34.2385, 54) -> (27.5928, 51) centre (31.5928, 51) ccw
  line L26 (34.2385, 54) -> (35.947, 54)
  arc A33 (42.5928, 51) -> (35.947, 54) centre (38.5928, 51) ccw
  line L27 (42.5928, 51) -> (42.5928, 48)
  arc A34 (35.947, 45) -> (42.5928, 48) centre (38.5928, 48) ccw
  line L28 (35.947, 45) -> (34.2385, 45)
  arc A35 (27.5928, 48) -> (34.2385, 45) centre (31.5928, 48) ccw
  line L29 (42.5928, 51) -> (47.5928, 51)
  line L30 (47.5928, 51) -> (47.5928, 48)
  line L31 (47.5928, 48) -> (42.5928, 48)
  line L32 (42.5928, 48) -> (42.5928, 51)
  line L33 (27.5928, 51) -> (22.5928, 51)
  line L34 (22.5928, 51) -> (22.5928, 48)
  line L35 (22.5928, 48) -> (27.5928, 48)
  line L36 (27.5928, 48) -> (27.5928, 51)
  circle A36 centre (26.5928, 48) radius 1
  circle A37 centre (43.5928, 48) radius 1
  circle A38 centre (26.5928, 48) radius 4
  circle A39 centre (43.5928, 48) radius 4
  line L37 (-33.9001, 48) -> (-18.9001, 48)
  line L38 (-18.9001, 48) -> (-18.9001, 45)
  line L39 (-18.9001, 45) -> (-33.9001, 45)
  line L40 (-33.9001, 45) -> (-33.9001, 48)
  line L41 (-28.9001, 48) -> (-23.9001, 48)
  line L42 (-21.9001, 48) -> (-21.9001, 51)
  line L43 (-23.9001, 51) -> (-28.9001, 51)
  line L44 (-30.9001, 51) -> (-30.9001, 48)
  line L45 (-26.4001, 51) -> (-26.4001, 125.4272)
  arc A40 (-28.9001, 51) -> (-30.9001, 51) centre (-29.9001, 51) ccw
  arc A41 (-21.9001, 51) -> (-23.9001, 51) centre (-22.9001, 51) ccw
  arc A42 (-30.9001, 48) -> (-28.9001, 48) centre (-29.9001, 48) ccw
  arc A43 (-23.9001, 48) -> (-21.9001, 48) centre (-22.9001, 48) ccw
  line L46 (-33.9001, 48) -> (-33.9001, 51)
  arc A44 (-27.2544, 54) -> (-33.9001, 51) centre (-29.9001, 51) ccw
  line L47 (-27.2544, 54) -> (-25.5459, 54)
  arc A45 (-18.9001, 51) -> (-25.5459, 54) centre (-22.9001, 51) ccw
  line L48 (-18.9001, 51) -> (-18.9001, 48)
  arc A46 (-25.5459, 45) -> (-18.9001, 48) centre (-22.9001, 48) ccw
  line L49 (-25.5459, 45) -> (-27.2544, 45)
  arc A47 (-33.9001, 48) -> (-27.2544, 45) centre (-29.9001, 48) ccw
  line L50 (-18.9001, 51) -> (-13.9001, 51)
  line L51 (-13.9001, 51) -> (-13.9001, 48)
  line L52 (-13.9001, 48) -> (-18.9001, 48)
  line L53 (-18.9001, 48) -> (-18.9001, 51)
  line L54 (-33.9001, 51) -> (-38.9001, 51)
  line L55 (-38.9001, 51) -> (-38.9001, 48)
  line L56 (-38.9001, 48) -> (-33.9001, 48)
  line L57 (-33.9001, 48) -> (-33.9001, 51)
  circle A48 centre (-34.9001, 48) radius 1
  circle A49 centre (-17.9001, 48) radius 1
  circle A50 centre (-34.9001, 48) radius 4
  circle A51 centre (-17.9001, 48) radius 4
  line L58 (-13.9001, 51) -> (22.5928, 51)
  line L59 (22.5928, 51) -> (22.5928, 48)
  line L60 (22.5928, 48) -> (-13.9001, 48)
  line L61 (-13.9001, 48) -> (-13.9001, 51)
  arc A52 (6.5669, 102.7056) -> (14.253, 93.0788) centre (13.05, 100) ccw projected
  line L62 (-18.5628, 119.1212) -> (-16.4155, 116.7864) projected
  point P0 (0, 0)
  point P1 (35.0928, 48)
  point P2 (-26.4001, 48)
  point P3 (-16.9001, 48)
  point P4 (25.5928, 48)
  point P5 (44.5928, 48)
  point P6 (46.2385, 51)
  point P7 (42.5018, 51.8483)
  point P8 (41.4891, 53.7588)
  point P9 (39.2667, 51.7388)
  point P10 (30.9189, 51.7388)
  point P11 (28.6964, 53.7588)
  point P12 (27.6838, 51.8483)
  point P13 (23.947, 51)
  point P14 (-15.2544, 51)
  point P15 (-18.9911, 51.8483)
  point P16 (-33.8091, 51.8483)
  point P17 (-37.5459, 51)
  point P18 (-35.9001, 48)
  dimension "d38" = 15
  dimension "d39" = 9
  dimension "d40" = 15
  dimension "d41" = 3
  dimension "d42" = 9
  dimension "d43" = 3
  dimension "d44" = 2
  dimension "d45" = 2
  dimension "d46" = 2
  dimension "d47" = 2
  dimension "d48" = 4.5
  dimension "d50" = 4.5
  dimension "d51" = 3
  dimension "d52" = 5
  dimension "d53" = 3
  dimension "d54" = 5
  dimension "d55" = 3
  dimension "d56" = 2
  dimension "d57" = 2
  dimension "d58" = 3
  dimension "d59" = 3
  dimension "d61" = 15
  dimension "d62" = 3
  dimension "d63" = 9
  dimension "d64" = 3
  dimension "d65" = 2
  dimension "d66" = 2
  dimension "d67" = 2
  dimension "d68" = 2
  dimension "d69" = 4.5
  dimension "d70" = 4.5
  dimension "d71" = 3
  dimension "d72" = 5
  dimension "d73" = 3
  dimension "d74" = 5
  dimension "d75" = 3
  dimension "d76" = 2
  dimension "d77" = 2
  dimension "d78" = 3
  dimension "d79" = 3
  constraints: 92 end point, 32 point on circle, 24 centre point, 22 parallel, 16 point on line, 12 tangent, 11 perpendicular, 9 horizontal, 6 midpoint, 2 vertical, 1 coincident, 14 other
  measures "d38" distance of L0.start L0.end
  measures "d39" distance between parallel lines of L12 L13
  measures "d40" distance of L17.end L18.end
  measures "d41" distance of L16.end L17.end
  measures "d42" distance of L23.start L21.end
  measures "d43" distance of L21.end L21.start
  measures "d44" diameter of A28
  measures "d45" diameter of A29
  measures "d46" diameter of A30
  measures "d47" diameter of A31
  measures "d48" distance from line of L21 point (35.093, 48)
  measures "d50" distance between parallel lines of L21 L24
  measures "d51" distance between parallel lines of L23 L25
  measures "d52" distance of L30.end L31.end
  measures "d53" distance of L29.end L30.end
  measures "d54" distance of L35.end L34.end
  measures "d55" distance of L34.end L33.end
  measures "d56" diameter of A36
  measures "d57" diameter of A37
  measures "d58" radial gap between concentric circles of A36 A38
  measures "d59" radial gap between concentric circles of A37 A39
  measures "d61" distance of L39.start L40.start
  measures "d62" distance of L37.end L39.start
  measures "d63" distance of L44.start L42.end
  measures "d64" distance of L42.end L42.start
  measures "d65" diameter of A40
  measures "d66" diameter of A41
  measures "d67" diameter of A42
  measures "d68" diameter of A43
  measures "d69" distance from line of L42 point (-26.4, 48)
  measures "d70" distance between parallel lines of L42 L45
  measures "d71" distance between parallel lines of L44 L46
  measures "d72" distance of L52.start L53.start
  measures "d73" distance of L50.end L52.start
  measures "d74" distance of L57.start L55.end
  measures "d75" distance of L55.end L55.start
  measures "d76" diameter of A48
  measures "d77" diameter of A49
  measures "d78" radial gap between concentric circles of A48 A50
  measures "d79" radial gap between concentric circles of A49 A51
extrude "押し出し4" add sketch "スケッチ4" against normal blind 3 contours L60 L51 L58 L12 | L60 L13 L58 L34 | A38 L33 L25 A36 L35 | L34 L33 A38 | L12 L58 L13 L60 | A51 L50 L51 | L52 A49 L48 L50 A51 | A38 A32 L33 | A35 L1 A38 L18 | L18 L19 A35 | L18 A38 A30 L1 A31 A39 | L50 A45 A51 | A32 A38 L1 L25 | A32 A11 A28 L23 A38 | A46 L39 A51 L37 | L37 A51 A45 L48 | L38 L39 A46 | A51 L42 A41 L43 L45 L47 A45 | L39 A50 A42 L37 A43 A51 | A39 L1 L16 A34 L18 | A34 L17 L18 | A39 A33 L27 L16 L1 | L21 A29 A11 A33 A39 | A39 L29 L30 | L31 A37 L27 L29 A39 | L45 L43 A40 L44 A50 A44 L47 | L39 A47 L37 A50 | A39 L29 A33 | L39 L40 A47 | L37 L46 A44 A50 | A50 L54 L46 A48 L56 | L55 L54 A50 | A44 L54 A50
extrude "押し出し5" cut sketch "スケッチ4" against normal blind 10 contours A28 L22 A29 A11
sketch "スケッチ5" plane through (0, 0, -3) normal (0, 0, -1) x (-1, 0, 0)
  arc A0 (39.5928, 51) -> (37.5928, 51) centre (38.5928, 51) ccw projected
  line L0 (39.5928, 51) -> (39.5928, 48) projected
  arc A1 (37.5928, 48) -> (39.5928, 48) centre (38.5928, 48) ccw projected
  line L1 (37.5928, 48) -> (32.5928, 48) projected
  arc A2 (30.5928, 48) -> (32.5928, 48) centre (31.5928, 48) ccw projected
  line L2 (30.5928, 48) -> (30.5928, 51) projected
  arc A3 (32.5928, 51) -> (30.5928, 51) centre (31.5928, 51) ccw projected
  line L3 (32.5928, 51) -> (37.5928, 51) projected
  arc A4 (41.4891, 53.7588) -> (33.4453, 66.3922) centre (35.0928, 58.5637) ccw projected
  arc A5 (32.3566, 66.9011) -> (33.4453, 66.3922) centre (33.2394, 67.3708) ccw projected
  line L4 (32.3566, 66.9011) -> (17.9557, 93.9721) projected
  arc A6 (18.1172, 95.1344) -> (17.9557, 93.9721) centre (18.8385, 94.4418) ccw projected
  arc A7 (18.1172, 95.1344) -> (9.4271, 106.0187) centre (13.05, 100) ccw projected
  arc A8 (8.2579, 106.1185) -> (9.4271, 106.0187) centre (8.9114, 106.8755) ccw projected
  line L5 (8.2579, 106.1185) -> (-4.9702, 117.5381) projected
  arc A9 (-5.288, 118.533) -> (-4.9702, 117.5381) centre (-4.3167, 118.295) ccw projected
  arc A10 (-5.288, 118.533) -> (-12.7725, 122.8527) centre (-9.6587, 119.604) ccw projected
  arc A11 (-13.793, 122.6301) -> (-12.7725, 122.8527) centre (-13.4645, 123.5746) ccw projected
  line L6 (-13.793, 122.6301) -> (-17.7414, 124.0035) projected
  arc A12 (-18.4115, 125.0013) -> (-17.7414, 124.0035) centre (-17.4129, 124.948) ccw projected
  arc A13 (-18.4115, 125.0013) -> (-22.8335, 118.2662) centre (-26.4001, 125.4272) ccw projected
  arc A14 (-21.6516, 118.048) -> (-22.8335, 118.2662) centre (-22.3876, 117.3711) ccw projected
  line L7 (-21.6516, 118.048) -> (28.1361, 63.912) projected
  arc A15 (28.2548, 62.7161) -> (28.1361, 63.912) centre (27.4001, 63.2351) ccw projected
  arc A16 (28.2548, 62.7161) -> (28.6964, 53.7588) centre (35.0928, 58.5637) ccw projected
  arc A17 (28.6964, 53.7588) -> (27.6838, 51.8483) centre (31.5928, 51) ccw projected
  arc A18 (27.6838, 51.8483) -> (23.947, 51) centre (26.5928, 48) ccw projected
  line L8 (23.947, 51) -> (-15.2544, 51) projected
  arc A19 (-15.2544, 51) -> (-18.9911, 51.8483) centre (-17.9001, 48) ccw projected
  arc A20 (-18.9911, 51.8483) -> (-25.5459, 54) centre (-22.9001, 51) ccw projected
  line L9 (-25.5459, 54) -> (-27.2544, 54) projected
  arc A21 (-27.2544, 54) -> (-33.8091, 51.8483) centre (-29.9001, 51) ccw projected
  arc A22 (-33.8091, 51.8483) -> (-37.5459, 51) centre (-34.9001, 48) ccw projected
  line L10 (-37.5459, 51) -> (-38.9001, 51) projected
  line L11 (-38.9001, 51) -> (-38.9001, 48) projected
  line L12 (-38.9001, 48) -> (-35.9001, 48) projected
  arc A23 (-33.9001, 48) -> (-35.9001, 48) centre (-34.9001, 48) ccw projected
  line L13 (-33.9001, 48) -> (-33.9001, 45) projected
  line L14 (-33.9001, 45) -> (-18.9001, 45) projected
  line L15 (-18.9001, 45) -> (-18.9001, 48) projected
  arc A24 (-16.9001, 48) -> (-18.9001, 48) centre (-17.9001, 48) ccw projected
  line L16 (-16.9001, 48) -> (25.5928, 48) projected
  arc A25 (27.5928, 48) -> (25.5928, 48) centre (26.5928, 48) ccw projected
  line L17 (27.5928, 48) -> (27.5928, 45) projected
  line L18 (27.5928, 45) -> (42.5928, 45) projected
  line L19 (42.5928, 45) -> (42.5928, 48) projected
  arc A26 (44.5928, 48) -> (42.5928, 48) centre (43.5928, 48) ccw projected
  line L20 (44.5928, 48) -> (47.5928, 48) projected
  line L21 (47.5928, 48) -> (47.5928, 51) projected
  line L22 (47.5928, 51) -> (46.2385, 51) projected
  arc A27 (46.2385, 51) -> (42.5018, 51.8483) centre (43.5928, 48) ccw projected
  arc A28 (42.5018, 51.8483) -> (41.4891, 53.7588) centre (38.5928, 51) ccw projected
  line L23 (-30.9001, 48) -> (-30.9001, 51) projected
  arc A29 (-28.9001, 51) -> (-30.9001, 51) centre (-29.9001, 51) ccw projected
  line L24 (-28.9001, 51) -> (-23.9001, 51) projected
  arc A30 (-21.9001, 51) -> (-23.9001, 51) centre (-22.9001, 51) ccw projected
  line L25 (-21.9001, 51) -> (-21.9001, 48) projected
  arc A31 (-23.9001, 48) -> (-21.9001, 48) centre (-22.9001, 48) ccw projected
  line L26 (-23.9001, 48) -> (-28.9001, 48) projected
  arc A32 (-30.9001, 48) -> (-28.9001, 48) centre (-29.9001, 48) ccw projected
  arc A33 (6.5669, 102.7056) -> (14.253, 93.0788) centre (13.05, 100) ccw projected
  arc A34 (15.3071, 92.5632) -> (14.253, 93.0788) centre (14.4242, 92.0935) ccw projected
  line L27 (15.3071, 92.5632) -> (24.5983, 75.0975) projected
  arc A35 (22.9794, 73.9509) -> (24.5983, 75.0975) centre (23.7154, 74.6278) ccw projected
  line L28 (22.9794, 73.9509) -> (-13.0309, 113.1062) projected
  line L29 (-16.4155, 116.7864) -> (-18.5628, 119.1212) projected
  arc A36 (-17.4982, 120.7426) -> (-18.5628, 119.1212) centre (-17.8267, 119.7981) ccw projected
  line L30 (-17.4982, 120.7426) -> (-14.7786, 119.7967) projected
  arc A37 (-14.1165, 118.9889) -> (-14.7786, 119.7967) centre (-15.1071, 118.8522) ccw projected
  arc A38 (-14.1165, 118.9889) -> (-13.9936, 118.3962) centre (-9.6587, 119.604) ccw projected
  arc A39 (-14.28, 117.3918) -> (-13.9936, 118.3962) centre (-14.9569, 118.1278) ccw projected
  line L31 (-14.28, 117.3918) -> (-15.0025, 116.7273) projected
  arc A40 (-16.4155, 116.7864) -> (-15.0025, 116.7273) centre (-15.6794, 117.4633) ccw projected
  circle A41 centre (35.0928, 58.5637) radius 4 projected
  circle A42 centre (-26.4001, 125.4272) radius 4 projected
  circle A43 centre (13.05, 100) radius 4.025 projected
  circle A44 centre (-9.6587, 119.604) radius 1.5 projected
  arc A45 (-12.9717, 114.5191) -> (-13.0309, 113.1062) centre (-12.2948, 113.7831) ccw projected
  line L32 (-12.9717, 114.5191) -> (-12.2492, 115.1836) projected
  arc A46 (-11.2244, 115.3851) -> (-12.2492, 115.1836) centre (-11.5723, 114.4476) ccw projected
  arc A47 (-11.2244, 115.3851) -> (-7.9613, 115.4364) centre (-9.6587, 119.604) ccw projected
  arc A48 (-6.9306, 115.2672) -> (-7.9613, 115.4364) centre (-7.5841, 114.5103) ccw projected
  line L33 (-6.9306, 115.2672) -> (6.2975, 103.8477) projected
  arc A49 (6.5669, 102.7056) -> (6.2975, 103.8477) centre (5.644, 103.0907) ccw projected
  line L34 (-26.4001, 125.4272) -> (-26.4001, 51) construction
  line L35 (-27.9001, 125.4272) -> (-27.9001, 51)
  line L36 (-24.9001, 51) -> (-24.9001, 125.4272)
  arc A50 (-24.9001, 125.4272) -> (-27.9001, 125.4272) centre (-26.4001, 125.4272) ccw
  arc A51 (-27.9001, 51) -> (-24.9001, 51) centre (-26.4001, 51) ccw
  circle A52 centre (13.05, 100) radius 4.025 projected
  line L37 (13.05, 100) -> (-26.4001, 51) construction
  line L38 (11.8816, 100.9407) -> (-27.5685, 51.9407)
  line L39 (-25.2317, 50.0593) -> (14.2184, 99.0593)
  arc A53 (14.2184, 99.0593) -> (11.8816, 100.9407) centre (13.05, 100) ccw
  arc A54 (-27.5685, 51.9407) -> (-25.2317, 50.0593) centre (-26.4001, 51) ccw
  point P0 (0, 0)
  point P1 (-26.4001, 88.2136)
  point P2 (-6.6751, 75.5)
  point P3 (-21.4676, 54.7347)
  point P4 (5.6265, 88.3876)
  point P5 (3.5728, 90.6206)
  point P6 (-24.9001, 55.255)
  point P7 (-24.9001, 117.569)
  point P8 (-27.9001, 117.569)
  point P9 (-27.9001, 54.4641)
  point P10 (7.529, 90.7507)
  point P11 (9.9145, 93.7136)
  point P12 (7.5777, 95.5949)
  point P13 (5.4754, 92.9837)
  dimension "d84" = 3
  dimension "d85" = 3
  constraints: 16 end point, 8 point on circle, 8 tangent, 4 centre point, 3 midpoint, 2 parallel, 1 concentric
  measures "d84" diameter of A51
  measures "d85" diameter of A54
extrude "押し出し6" add sketch "スケッチ5" against normal blind 3 contours A13 L36 L38 L9 A21 L35 | L38 L7 L39 A20 L36 | L36 A20 L9 L38 | L38 A33 L39 L28
fillet "フィレット2" radius 1 21 edges at (21.4676, 54.7347, -1.5) (-5.6265, 88.3876, -1.5) (-3.5728, 90.6206, -1.5) (24.9001, 55.255, -1.5) (24.9001, 117.569, -1.5) (27.9001, 117.569, -1.5) (27.9001, 54.4641, -1.5) (-7.5777, 95.5949, -1.5) (-5.4754, 92.9837, -1.5) (-7.529, 90.7507, -1.5) (-9.9145, 93.7136, -1.5) (18.9911, 51.8483, -1.5) (-46.2385, 51, -1.5) (-42.5018, 51.8483, -1.5) (-41.4891, 53.7588, -1.5) (-28.6964, 53.7588, -1.5) (-27.6838, 51.8483, -1.5) (-23.947, 51, -1.5) (15.2544, 51, -1.5) (33.8091, 51.8483, -1.5) (37.5459, 51, -1.5)